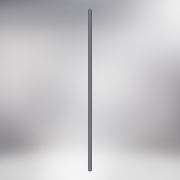
# Autodesk Inventor part: Part1
Saved by Autodesk Inventor 2016 (Build 200138000, 138)
## iProperties
Created: 2015-05-20
Part Number: Part1
Material: Generic
Document SubType Name: Modeling
Designer: as
Mass: 20.1062 g
Surface Area: 101.536 cm^2
Volume: 20.1062 cm^3
Density: 1 g/cm^3
Appearance: Default
Author: as
Autodesk Inventor part; units mm, degrees
ref_plane "YZ Plane" through (0, 0, 0) normal (1, 0, 0) x (0, 1, 0)
ref_plane "XZ Plane" through (0, 0, 0) normal (0, 1, 0) x (-1, 0, 0)
ref_plane "XY Plane" through (0, 0, 0) normal (0, 0, 1) x (1, 0, 0)
sketch "Sketch1" plane through (0, 0, 0) normal (0, 0, 1) x (1, 0, 0)
  circle A0 centre (0, 0) radius 4
  dimension "d0" = 400
  constraints: 1 centre point, 1 coincident
extrude "Extrusion1" add sketch "Sketch1" along normal blind 400
body "Solid1"
